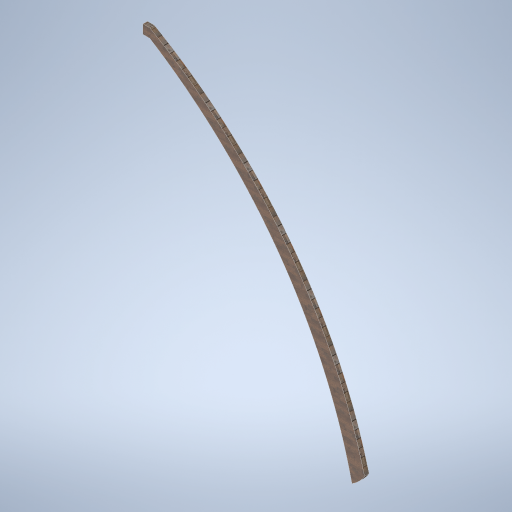
# Autodesk Inventor part: curve_beam_03
Saved by Autodesk Inventor 2024.2 (Build 282272000, 272)
## iProperties
Created: 2024-05-20
Part Number: curve_beam_03
Material: Wood (Maple)
Document SubType Name: Modeling
Designer: LOSTER_1
Density: 0.67 g/cm^3
Appearance: Natural Maple - Glossy Dark Tint
Author: LOSTER_1
Autodesk Inventor part; units mm, degrees
ref_plane "YZ Plane" through (0, 0, 0) normal (1, 0, 0) x (0, 1, 0)
ref_plane "XZ Plane" through (0, 0, 0) normal (0, 1, 0) x (-1, 0, 0)
ref_plane "XY Plane" through (0, 0, 0) normal (0, 0, 1) x (1, 0, 0)
sketch "Sketch1" plane through (0, 0, 0) normal (0, 0, 1) x (1, 0, 0)
  ellipse E0 centre (4015.7888, -1667.4861) end of major axis (4015.7888, -2467.4861) minor radius 800 (4424.4298, -2355.2452) -> (4701.6709, -2079.2696) ccw
  arc A0 (4701.6709, -2079.2696) -> (-25.36, 4106.1752) centre (-4980.6691, -4579.7278) ccw
  arc A1 (4424.4298, -2355.2452) -> (-25.36, 3906.647) centre (-5326.6573, -4572.5185) ccw
  arc A2 (4424.4298, -2355.2452) -> (4701.6709, -2079.2696) centre (4015.7888, -1667.4861) ccw
  line L0 (-25.36, 4106.1752) -> (-175.36, 4106.1752)
  line L1 (-175.36, 4106.1752) -> (-175.36, 3906.647)
  line L2 (-175.36, 3906.647) -> (-25.36, 3906.647)
  point P0 (0, 0)
  dimension "d0" = 10000
  dimension "d1" = 10000
  dimension "d2" = 150
  constraints: 6 end point, 6 point on circle, 3 centre point, 2 perpendicular, 1 horizontal, 4 other
  measures "d0" radius of A0
  measures "d1" radius of A1
  measures "d2" distance of L0.start L0.end
extrude "Extrusion1" add sketch "Sketch1" along normal blind 100
body "Solid1"
